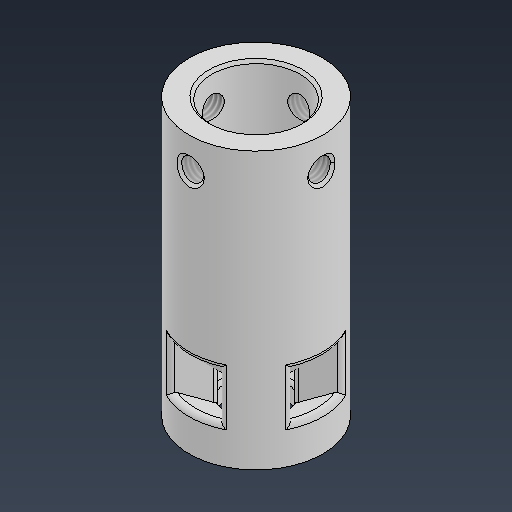
# Autodesk Inventor part: Chamferer
Saved by Autodesk Inventor 2026.2 (Build 302298010, 298A)
## iProperties
Created: 2026-06-12
Part Number: Chamferer
Material: Generic
Document SubType Name: Modeling
Designer: szymo
Density: 1 g/cm^3
Appearance: Default
Author: szymo
Autodesk Inventor part; units mm, degrees
ref_plane "YZ Plane" through (0, 0, 0) normal (1, 0, 0) x (0, 1, 0)
ref_plane "XZ Plane" through (0, 0, 0) normal (0, 1, 0) x (-1, 0, 0)
ref_plane "XY Plane" through (0, 0, 0) normal (0, 0, 1) x (1, 0, 0)
sketch "Sketch1" plane through (0, 0, 0) normal (1, 0, 0) x (0, 1, 0)
  line L0 (0, 0) -> (0, -3.2) construction
  line L1 (0, -3.2) -> (-5.2, -3.2)
  line L2 (-5.2, -3.2) -> (-5.2, -7.5)
  line L3 (-5.2, -7.5) -> (25.8, -7.5)
  line L4 (38.8, -3.2) -> (0, -3.2) construction
  line L5 (0, 0) -> (-5.2, 0) construction
  line L6 (0, -3.2) -> (-3.2, 0) construction
  line L7 (-5.2, -3.2) -> (-5.2, 0)
  line L8 (0, -3.2) -> (4.8, -3.2)
  line L9 (4.8, -3.2) -> (4.8, -4.95)
  line L10 (4.8, -4.95) -> (25.8, -4.95)
  line L11 (25.8, -4.95) -> (25.8, -3.2)
  line L12 (25.8, -7.5) -> (25.8, -3.2)
  line L13 (25.8, -4.95) -> (25.8, -4.95)
  dimension "d0" = 3.2
  dimension "d1" = 45
  dimension "d2" = 2
  dimension "d3" = 5.2
  dimension "d4" = 4.8
  dimension "d5" = 21
  dimension "d6" = 42
  dimension "d7" = 4.95
  dimension "d8" = 0
  dimension "d9" = 7.5
  dimension "d11" = 2.55
  dimension "d12" = 13
  constraints: 28 end point, 6 point on line, 5 perpendicular, 3 vertical, 2 horizontal, 1 collinear
  measures "d0" distance of L0.start L0.end
  measures "d1" angle of L5 L6
  measures "d2" distance of L5.end L6.end
  measures "d3" distance from line of L7 L0.start
  measures "d4" distance from line of L0.end L9
  measures "d5" distance of L9.end L10.end
  measures "d6" horizontal distance of L4.start L6.end
  measures "d7" distance from line of L10 L6.end
  measures "d8" distance between parallel lines of L12 L11
  measures "d9" distance from line of L3 L5.end
  measures "d11" distance between parallel lines of L10 L3
  measures "d12" distance from line of L4.start L12
revolve "Revolution1" add sketch "Sketch1" angle 360 about axis through (0, 0, 0) along (0, -1, 0)
sketch "Sketch2" plane through (0, 0, 0) normal (1, 0, 0) x (0, 1, 0)
  line L0 (25.8, 7.5) -> (25.8, -7.5) projected
  line L1 (-5.2, 7.5) -> (-5.2, -7.5) projected
  line L2 (25.8, 7.5) -> (25.8, -7.5) projected
  line L3 (25.8, 0) -> (22.3, 0)
  point P0 (0, 0)
  dimension "d44" = 3.5
  constraints: 2 end point, 1 horizontal, 1 midpoint
  measures "d44" distance of L3.start L3.end
hole "Hole1" at (0, 22.3, 0) direction (-1, 0, 0) diameter 2.459 depth 10.05 thread size "M3x0.5" class "6H" standard "ISO Metric profile"
sketch "Sketch3" plane through (0, 0, 0) normal (1, 0, 0) x (0, 1, 0)
  line L0 (4.8, 4.95) -> (4.8, -4.95) projected
  line L1 (-5.2, -3.2) -> (4.8, -3.2) projected
  line L2 (-5.2, 3.2) -> (4.8, 3.2) projected
  line L3 (25.8, -7.5) -> (-5.2, -7.5) projected
  line L4 (25.8, 7.5) -> (-5.2, 7.5) projected
  line L5 (-3.2, -3.2) -> (-0.7174, -7.5)
  line L6 (4.8, 0) -> (0.3696, 0) construction
  line L7 (4.5216, -7.5) -> (0.2216, -3.2)
  point P0 (0, 0)
  dimension "d32" = 60
  dimension "d33" = 2
  dimension "d34" = 45
  dimension "d35" = 2
  constraints: 6 end point, 4 point on line, 1 horizontal, 1 midpoint
  measures "d32" angle of L5 L1
  measures "d33" distance of L1.start L5.start
  measures "d34" angle of L7 L1
  measures "d35" distance from line of L7 L0.end
revolve "Revolution2" cut sketch "Sketch3" angle 45 mid plane about axis through (0, 4.8, 0) along (0, -1, 0)
fillet "Fillet1" radius 0.5 12 edges at (0.6243, 0.2216, -3.1385) (-0.6243, 0.2216, -3.1385) (1.2246, -1.4892, -2.9564) (-1.2246, -1.4892, -2.9564) (0.6243, -3.2, -3.1385) (-0.6243, -3.2, -3.1385) (1.4632, 4.5216, -7.3559) (-1.4632, 4.5216, -7.3559) (2.8701, 1.9021, -6.9291) (-2.8701, 1.9021, -6.9291) (1.4632, -0.7174, -7.3559) (-1.4632, -0.7174, -7.3559)
pattern_circular "Circular Pattern1" count 4 over 360 about axis through (0, -10, 0) along (0, 1, 0) of "Revolution2", "Fillet1", "Hole1"
chamfer "Chamfer2" distance 0.3 angle 45 7 edges at (-7.3985, 22.2977, 1.2295) (1.2295, 22.3004, 7.3985) (7.3985, 22.2977, -1.2295) (0.9177, 21.4818, -7.4436) (0.9197, 23.116, -7.4434) (-1.2295, 22.2999, -7.3985) (0, 25.8, 4.95)
body "Solid1"
